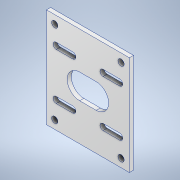
# Autodesk Inventor part: Neo Mounting Plate
Saved by Autodesk Inventor 2020 (Build 240168000, 168)
## iProperties
Created: 2020-02-02
Part Number: Neo Mounting Plate
Material: Aluminum 6061
Document SubType Name: Modeling
Designer: JimAndVal
Density: 2.7 g/cm^3
Appearance: Aluminum - Flat
Author: JimAndVal
Autodesk Inventor part; units mm, degrees
ref_plane "YZ Plane" through (0, 0, 0) normal (1, 0, 0) x (0, 1, 0)
ref_plane "XZ Plane" through (0, 0, 0) normal (0, 1, 0) x (-1, 0, 0)
ref_plane "XY Plane" through (0, 0, 0) normal (0, 0, 1) x (1, 0, 0)
sketch "Neo Motor Mount" plane through (0, 0, 0) normal (0, 0, 1) x (1, 0, 0)
  line L0 (-58.0667, 162.6468) -> (-53.1939, 138.405) construction
  line L1 (-57.5073, 159.8642) -> (-45.1815, 162.9896)
  line L2 (-53.7533, 141.1877) -> (-41.4275, 144.3131)
  arc A0 (-57.5073, 159.8642) -> (-52.8309, 141.4216) centre (-55.6303, 150.5259) ccw
  arc A1 (-46.2915, 152.4) -> (-46.438, 153.0215) centre (-55.6303, 150.5259) ccw
  arc A2 (-49.53, 157.8411) -> (-51.2107, 158.9635) centre (-55.6303, 150.5259) ccw
  arc A3 (-52.747, 152.4) -> (-52.6427, 151.7743) centre (-43.3045, 153.6514) ccw
  arc A4 (-49.53, 160.8603) -> (-51.2107, 158.9635) centre (-43.3045, 153.6514) ccw
  arc A5 (-41.4275, 144.3131) -> (-46.1039, 162.7557) centre (-43.3045, 153.6514) ccw
  line L3 (-30.6788, 181.9654) -> (-23.3726, 145.6169) construction
  line L4 (-43.3455, 180.5359) -> (-35.6081, 142.0424) construction
  arc A6 (-42.1579, 174.6277) -> (-41.2194, 169.9586) centre (-41.6886, 172.2931) ccw
  line L5 (-35.6081, 142.0424) -> (-32.6003, 127.0788) construction
  line L6 (-23.3726, 145.6169) -> (-20.1494, 129.5815) construction
  arc A7 (-35.0803, 139.4164) -> (-34.1417, 134.7473) centre (-34.611, 137.0818) ccw
  arc A8 (-21.6908, 137.25) -> (-22.6293, 141.9191) centre (-22.16, 139.5845) ccw
  line L7 (-35.0803, 139.4164) -> (-22.6293, 141.9191)
  line L8 (-34.1417, 134.7473) -> (-21.6908, 137.25)
  arc A9 (-77.3692, 167.55) -> (-76.4307, 162.8809) centre (-76.9, 165.2155) ccw
  arc A10 (-63.9797, 165.3836) -> (-64.9183, 170.0527) centre (-64.449, 167.7182) ccw
  arc A11 (-70.2916, 132.3387) -> (-69.3531, 127.6696) centre (-69.8223, 130.0042) ccw
  arc A12 (-56.9021, 130.1723) -> (-57.8406, 134.8414) centre (-57.3714, 132.5069) ccw
  line L9 (-70.2916, 132.3387) -> (-57.8406, 134.8414)
  line L10 (-69.3531, 127.6696) -> (-56.9021, 130.1723)
  line L11 (-77.3692, 167.55) -> (-64.9183, 170.0527)
  line L12 (-76.4307, 162.8809) -> (-63.9797, 165.3836)
  arc A13 (-28.7684, 172.4613) -> (-29.7069, 177.1304) centre (-29.2377, 174.7958) ccw
  line L13 (-42.1579, 174.6277) -> (-29.7069, 177.1304)
  line L14 (-41.2194, 169.9586) -> (-28.7684, 172.4613)
  line L15 (-45.711, 165.6236) -> (-40.743, 140.9077) construction
  dimension "d0" = 4.7625
  dimension "d1" = 4.7625
  dimension "d2" = 4.7625
  dimension "d3" = 4.7625
  dimension "d4" = 4.7625
  dimension "d5" = 4.7625
  dimension "d6" = 4.7625
  dimension "d7" = 4.7625
  dimension "d8" = 24.7159
  measures "d0" diameter of A6
  measures "d1" diameter of A7
  measures "d2" diameter of A8
  measures "d3" diameter of A9
  measures "d4" diameter of A10
  measures "d5" diameter of A11
  measures "d6" diameter of A12
  measures "d7" diameter of A13
  measures "d8" vertical distance of L15.start L15.end
sketch "Sketch2" plane through (0, 0, 0) normal (0, 0, 1) x (1, 0, 0)
  line L0 (-17.9578, 11.9804) -> (-17.9578, -15.3576) construction
  line L1 (-6.35, 10.8428) -> (-6.35, -16.1397) construction
  line L2 (-24.3078, 11.5893) -> (-24.3078, -16.1397) construction
  line L3 (-26.7514, 17.9578) -> (24.334, 17.9578) construction
  line L4 (-24.3078, 11.5893) -> (-24.3078, 20.3391) construction
  line L5 (-17.9578, 11.9804) -> (-17.9578, 19.9735) construction
  arc A0 (-24.3078, 20.3391) -> (-24.3078, 15.5765) centre (-24.3078, 17.9578) ccw
  line L6 (-11.6078, 11.5893) -> (-11.6078, -16.1397) construction
  line L7 (-11.6078, 11.5893) -> (-11.6078, 20.3391) construction
  arc A1 (-11.6078, 15.5765) -> (-11.6078, 20.3391) centre (-11.6078, 17.9578) ccw
  line L8 (-24.3078, 20.3391) -> (-11.6078, 20.3391)
  line L9 (-24.3078, 15.5765) -> (-11.6078, 15.5765)
  line L10 (0, 0) -> (0, 28.3511) construction
  arc A2 (24.3078, 15.5765) -> (24.3078, 20.3391) centre (24.3078, 17.9578) ccw
  arc A3 (11.6078, 20.3391) -> (11.6078, 15.5765) centre (11.6078, 17.9578) ccw
  line L11 (24.3078, 20.3391) -> (11.6078, 20.3391)
  line L12 (24.3078, 15.5765) -> (11.6078, 15.5765)
  arc A4 (-6.35, 9.525) -> (-6.35, -9.525) centre (-6.35, 0) ccw
  arc A5 (6.35, -9.525) -> (6.35, 9.525) centre (6.35, 0) ccw
  line L13 (-6.35, 0) -> (-37.1588, 0) construction
  line L14 (-26.7514, -17.9578) -> (24.334, -17.9578) construction
  arc A6 (-24.3078, -15.5765) -> (-24.3078, -20.3391) centre (-24.3078, -17.9578) ccw
  arc A7 (-11.6078, -20.3391) -> (-11.6078, -15.5765) centre (-11.6078, -17.9578) ccw
  line L15 (-24.3078, -20.3391) -> (-11.6078, -20.3391)
  line L16 (-24.3078, -15.5765) -> (-11.6078, -15.5765)
  arc A8 (24.3078, -20.3391) -> (24.3078, -15.5765) centre (24.3078, -17.9578) ccw
  line L17 (24.3078, -20.3391) -> (11.6078, -20.3391)
  arc A9 (11.6078, -15.5765) -> (11.6078, -20.3391) centre (11.6078, -17.9578) ccw
  line L18 (24.3078, -15.5765) -> (11.6078, -15.5765)
  line L19 (-6.35, 9.525) -> (6.35, 9.525)
  line L20 (-6.35, -9.525) -> (6.35, -9.525)
  line L21 (31.75, -38.1) -> (-31.75, -38.1)
  line L22 (-31.75, -38.1) -> (-31.75, 38.1)
  line L23 (-31.75, 38.1) -> (31.75, 38.1)
  line L24 (31.75, 38.1) -> (31.75, -38.1)
  line L25 (31.75, -38.1) -> (-31.75, 38.1) construction
  line L26 (-31.75, -38.1) -> (31.75, 38.1) construction
  circle A10 centre (-25.4, 31.75) radius 2.3813
  circle A11 centre (25.4, 31.75) radius 2.3813
  circle A12 centre (-25.4, -31.75) radius 2.3813
  circle A13 centre (25.4, -31.75) radius 2.3813
  point P0 (-17.9578, -19.9735)
  dimension "d27" = 17.9578
  dimension "d28" = 6.35
  dimension "d29" = 6.35
  dimension "d31" = 17.9578
  dimension "d32" = 4.7625
  dimension "d33" = 19.05
  dimension "d34" = 63.5
  dimension "d35" = 76.2
  dimension "d36" = 4.7625
  dimension "d37" = 6.35
  dimension "d38" = 6.35
  constraints: 55 end point, 29 symmetric about line, 20 point on circle, 14 centre point, 6 point on line, 6 vertical, 5 horizontal, 2 midpoint, 2 parallel, 2 perpendicular, 2 tangent, 11 other
  measures "d27" distance from line of L10.start L0
  measures "d28" distance from line of L10.start L1
  measures "d29" distance between parallel lines of L0 L2
  measures "d31" distance from line of L10.start L3
  measures "d32" diameter of A0
  measures "d33" diameter of A4
  measures "d34" distance of L22.end L23.end
  measures "d35" distance of L21.start L23.end
  measures "d36" diameter of A10
  measures "d37" horizontal distance of L22.end A10.centre
  measures "d38" horizontal distance of L22.end A10.centre
extrude "Extrusion1" add sketch "Sketch2" along normal mid plane 3.175
body "Solid1"
